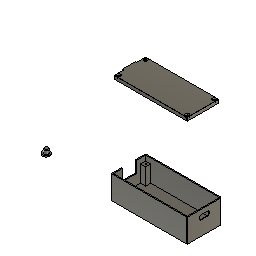
usb-relay (Autodesk Fusion 360 design; units mm, degrees)
Autodesk Fusion 360 part; units mm, degrees
note: some values were not read from the file. Set by a fixed rule: which sketch regions a step uses.
sketch "Skizze1" plane through (0, 0, 0) normal (0, 0, 1) x (1, 0, 0)
  line L0 (0, 0) -> (70, 0)
  line L1 (70, 0) -> (70, 30)
  line L2 (70, 30) -> (0, 30)
  line L3 (0, 30) -> (0, 0)
  circle A0 centre (68, 28) radius 0.7
  circle A1 centre (68, 2) radius 0.7
  circle A2 centre (2, 2) radius 0.7
  circle A3 centre (2, 28) radius 0.7
  line L4 (70, 15) -> (0, 15) construction
  circle A4 centre (36.4, 15) radius 2.5
  dimension "d1" = 70
  dimension "d2" = 30
  dimension "d3" = 1.4
  dimension "d4" = 2
  dimension "d5" = 2
  dimension "d6" = 1.4
  dimension "d7" = 2
  dimension "d8" = 1.4
  dimension "d9" = 2
  dimension "d10" = 1.4
  dimension "d29" = 5
  dimension "d54" = 36.4
  constraint horizontal L0
  constraint vertical L1
  constraint horizontal L2
  constraint vertical L3
  constraint coincident L0.start L3.end
  constraint vertical A0.centre A1.centre
  constraint horizontal A1.centre A2.centre
  constraint vertical A2.centre A3.centre
  constraint horizontal A0.centre A3.centre
  constraint perpendicular L1 L4
  constraint midpoint L3 L4.end
  measures "d1" distance of L0.start L0.end
  measures "d2" distance of L0.start L2.end
  measures "d3" diameter of A0
  measures "d4" distance of L1 A0.centre
  measures "d5" distance of L2 A0.centre
  measures "d6" diameter of A1
  measures "d7" distance of L0 A1.centre
  measures "d8" diameter of A2
  measures "d9" distance of L3 A2.centre
  measures "d10" diameter of A3
  measures "d29" diameter of A4
  measures "d54" distance of L3 A4.centre
extrude "Extrusion1" add sketch "Skizze1" against normal blind 1.6 contours L0 L1 L2 L3 | A4 makes body 1
sketch "Skizze2" plane through (0, 0, 0) normal (-1, 0, 0) x (0, -1, 0)
  line L0 (0, 0) -> (-30, 0)
  line L1 (-30, 0) -> (-30, -1.6)
  line L2 (-30, -1.6) -> (0, -1.6)
  line L3 (0, -1.6) -> (0, 0)
  line L4 (-17.85, 3.3) -> (-12.15, 3.3) construction
  line L5 (-12.15, 0) -> (-17.85, 0)
  arc A0 (-17.85, 3.3) -> (-19.5, 1.65) centre (-17.85, 1.65) ccw construction
  arc A1 (-19.5, 1.65) -> (-17.85, 0) centre (-17.85, 1.65) ccw construction
  arc A2 (-10.5, 1.65) -> (-12.15, 3.3) centre (-12.15, 1.65) ccw construction
  arc A3 (-12.15, 0) -> (-10.5, 1.65) centre (-12.15, 1.65) ccw construction
  arc A4 (-17.85, 3.8) -> (-20, 1.65) centre (-17.85, 1.65) ccw
  arc A5 (-20, 1.65) -> (-17.85, -0.5) centre (-17.85, 1.65) ccw
  line L6 (-12.15, -0.5) -> (-17.85, -0.5)
  arc A6 (-12.15, -0.5) -> (-10, 1.65) centre (-12.15, 1.65) ccw
  arc A7 (-10, 1.65) -> (-12.15, 3.8) centre (-12.15, 1.65) ccw
  line L7 (-17.85, 3.8) -> (-12.15, 3.8)
  point P0 (-19.5, 3.3)
  point P1 (-10.5, 3.3)
  point P2 (-19.5, 0)
  point P3 (-15, 0)
  dimension "d13" = 9
  dimension "d14" = 3.3
  dimension "d15" = 1.65
  dimension "d16" = 1.65
  dimension "d17" = 1.65
  dimension "d18" = 1.65
  dimension "d55" = -0.5
  constraint horizontal L4
  constraint horizontal L5
  constraint coincident P0 L4
  constraint tangent L4 A0
  constraint coincident L5 P3
  constraint coincident P2 L5
  constraint tangent L5 A1
  constraint coincident A0.end A1.start
  constraint coincident P1 L4
  constraint tangent L4 A2
  constraint tangent L5 A3
  constraint coincident A2.start A3.end
  measures "d13" distance of P0 P1
  measures "d14" distance of P0 P2
  measures "d15" radius of A0
  measures "d16" radius of A1
  measures "d17" radius of A2
  measures "d18" radius of A3
extrude "Extrusion2" add sketch "Skizze2" along normal blind 10 contours L0 L5 A5 L6 A6 | L0 L5 A4 A5 A6 A7 L7 bodies 1
sketch "Skizze3" plane through (70, 0, 0) normal (1, 0, 0) x (0, 1, 0)
  line L0 (30, 0) -> (0, 0)
  line L1 (0, 0) -> (0, -1.6)
  line L2 (0, -1.6) -> (30, -1.6)
  line L3 (30, -1.6) -> (30, 0)
  line L4 (8.25, 0) -> (21.75, 0)
  line L5 (21.75, 0) -> (21.75, 6)
  line L6 (21.75, 6) -> (8.25, 6)
  line L7 (8.25, 6) -> (8.25, 0)
  point P0 (15, 0)
  dimension "d21" = 13.5
  dimension "d22" = 6
  constraint horizontal L4
  constraint vertical L5
  constraint horizontal L6
  constraint vertical L7
  constraint midpoint L4 P0
  measures "d21" distance of L4.start L4.end
  measures "d22" distance of L4.start L6.end
extrude "Extrusion3" add sketch "Skizze3" along normal blind 10 separate body contours L0 L4 L5 L6 L7 makes body 2
extrude "Extrusion4" add sketch "Skizze2" against normal blind 2 contours L0 L5 A5 L6 A6 | L0 L5 A4 A5 A6 A7 L7 bodies 1
extrude "Extrusion5" add sketch "Skizze3" against normal blind 2 contours L0 L4 L5 L6 L7 bodies 1 2
extrude "Extrusion6" add sketch "Skizze1" along normal blind 18.5 contours A4 bodies 1
sketch "Skizze4" plane through (0, 0, 0) normal (0, 0, 1) x (1, 0, 0)
  line L0 (116.2217, 0) -> (187.2217, 0)
  line L1 (187.2217, 0) -> (187.2217, 31)
  line L2 (187.2217, 31) -> (116.2217, 31)
  line L3 (116.2217, 31) -> (116.2217, 0)
  line L4 (115.2217, -1) -> (188.2217, -1)
  line L5 (188.2217, -1) -> (188.2217, 32)
  line L6 (188.2217, 32) -> (115.2217, 32)
  line L7 (115.2217, 32) -> (115.2217, -1)
  line L8 (116.2217, 0) -> (121.2217, 0)
  line L9 (121.2217, 0) -> (121.2217, 5)
  line L10 (121.2217, 5) -> (116.2217, 5)
  line L11 (116.2217, 5) -> (116.2217, 0)
  line L12 (187.2217, 0) -> (182.2217, 0)
  line L13 (182.2217, 0) -> (182.2217, 5)
  line L14 (182.2217, 5) -> (187.2217, 5)
  line L15 (187.2217, 5) -> (187.2217, 0)
  line L16 (187.2217, 31) -> (182.2217, 31)
  line L17 (182.2217, 31) -> (182.2217, 26)
  line L18 (182.2217, 26) -> (187.2217, 26)
  line L19 (187.2217, 26) -> (187.2217, 31)
  line L20 (116.2217, 31) -> (121.2217, 31)
  line L21 (121.2217, 31) -> (121.2217, 26)
  line L22 (121.2217, 26) -> (116.2217, 26)
  line L23 (116.2217, 26) -> (116.2217, 31)
  dimension "d32" = 71
  dimension "d33" = 31
  dimension "d34" = 1
  dimension "d39" = 5
  dimension "d40" = 5
  dimension "d41" = 5
  dimension "d42" = 5
  dimension "d43" = 5
  dimension "d44" = 5
  dimension "d45" = 5
  dimension "d46" = 5
  constraint horizontal L0
  constraint vertical L1
  constraint horizontal L2
  constraint vertical L3
  constraint horizontal L8
  constraint vertical L9
  constraint horizontal L10
  constraint vertical L11
  constraint horizontal L12
  constraint vertical L13
  constraint horizontal L14
  constraint vertical L15
  constraint horizontal L16
  constraint vertical L17
  constraint horizontal L18
  constraint vertical L19
  constraint horizontal L20
  constraint vertical L21
  constraint horizontal L22
  constraint vertical L23
  measures "d32" distance of L0.start L0.end
  measures "d33" distance of L0.start L2.end
  measures "d39" distance of L0.start L8.end
  measures "d40" distance of L0.start L10.end
  measures "d41" distance of L0.end L12.end
  measures "d42" distance of L0.end L14.end
  measures "d43" distance of L1.end L16.end
  measures "d44" distance of L1.end L18.end
  measures "d45" distance of L2.end L20.end
  measures "d46" distance of L2.end L22.end
extrude "Extrusion7" add sketch "Skizze4" along normal blind 2 separate body contours L0 L3 L8 L9 L10 L11 | L0 L1 L2 L3 L9 L10 L13 L14 L17 L18 L21 L22 | L0 L1 L12 L13 L14 L15 | L2 L3 L20 L21 L22 L23 | L1 L2 L16 L17 L18 L19 makes body 3
extrude "Extrusion8" add sketch "Skizze4" along normal blind 23 bodies 3
extrude "Extrusion9" add sketch "Skizze4" along normal blind 18 contours L0 L3 L8 L9 L10 L11 | L0 L1 L12 L13 L14 L15 | L2 L3 L20 L21 L22 L23 | L1 L2 L16 L17 L18 L19 bodies 3
extrude "Extrusion10" add sketch "Skizze1" along normal blind 5 contours A0 | A1 | A2 | A3 bodies 1
move_body "Verschieben1" bodies 1 to x (-1, 0, 0) y (0, 1, 0) z (0, 0, -1) at (186.75, 0.5, -6)
move_body "Verschieben2" bodies 1 to x (1, 0, 0) y (0, 1, 0) z (0, 0, 1) at (0, 0, 24)
combine "Kombinieren2" operation cut target body 3 tool bodies 1
sketch "Skizze5" plane through (115.2217, 0, 0) normal (-1, 0, 0) x (0, -1, 0)
  line L0 (-32, 0) -> (1, 0)
  line L1 (1, 0) -> (1, 23)
  line L2 (1, 23) -> (-32, 23)
  line L3 (-32, 23) -> (-32, 0)
  line L4 (-22.25, 18) -> (-8.75, 18)
  line L5 (-8.75, 18) -> (-8.75, 23)
  line L6 (-8.75, 23) -> (-22.25, 23)
  line L7 (-22.25, 23) -> (-22.25, 18)
  line L8 (-8.75, 12) -> (-22.25, 12)
  line L9 (-22.25, 12) -> (-22.25, 18)
  line L10 (-22.25, 18) -> (-8.75, 18)
  line L11 (-8.75, 18) -> (-8.75, 12)
  constraint horizontal L4
  constraint vertical L5
  constraint horizontal L6
  constraint vertical L7
  constraint coincident L2 L5.end
extrude "Extrusion11" cut sketch "Skizze5" against normal blind 5 contours L2 L4 L5 L6 L7 L10 bodies 3
chamfer "Fase1" distance 0.5 angle 45 8 edges at (115.2217, -1, 11.5) (115.2217, 32, 11.5) (115.2217, 15.5, 0) (151.7217, -1, 0) (188.2217, 15.5, 0) (188.2217, -1, 11.5) (188.2217, 32, 11.5) (151.7217, 32, 0) on bodies 3
chamfer "Fase2" distance 0.5 angle 45 4 edges at (187.2217, 10.5, 16.35) (187.2217, 15.5, 14.2) (187.2217, 20.5, 16.35) (187.2217, 15.5, 18.5) on bodies 3
chamfer "Fase3" distance 0.3 angle 45 2 edges at (115.7217, 8.75, 12) (115.7217, 22.25, 12) on bodies 3
ref_plane "Arbeitsebene1" through (0, 0, 105) normal (0, 0, 1) x (1, 0, 0)
sketch "Skizze7" plane through (0, 0, 105) normal (0, 0, 1) x (1, 0, 0)
sketch "Skizze8" plane through (0, 0, 105) normal (0, 0, 1) x (1, 0, 0)
  line L0 (116.2217, 0) -> (187.2217, 0) construction
  line L1 (115.2217, -1) -> (188.2217, -1)
  line L2 (116.2217, 31) -> (116.2217, 0) construction
  line L3 (115.2217, 32) -> (115.2217, -1)
  line L4 (187.2217, 31) -> (116.2217, 31) construction
  line L5 (188.2217, 32) -> (115.2217, 32)
  line L6 (121.2217, 31) -> (121.2217, 26) construction
  line L7 (121.2217, 26) -> (116.2217, 26) construction
  line L8 (121.2217, 5) -> (116.2217, 5) construction
  line L9 (121.2217, 0) -> (121.2217, 5) construction
  line L10 (182.2217, 0) -> (182.2217, 5) construction
  line L11 (182.2217, 5) -> (187.2217, 5) construction
  line L12 (187.2217, 0) -> (187.2217, 31) construction
  line L13 (188.2217, -1) -> (188.2217, 32)
  line L14 (182.2217, 26) -> (187.2217, 26) construction
  line L15 (182.2217, 31) -> (182.2217, 26) construction
  circle A0 centre (184.7217, 2.5) radius 1.2
  circle A1 centre (118.7217, 2.5) radius 1.2
  circle A2 centre (118.7217, 28.5) radius 1.2
  circle A3 centre (184.7217, 28.5) radius 1.2
  circle A4 centre (184.7217, 2.5) radius 1.85
  circle A5 centre (118.7217, 2.5) radius 1.85
  circle A6 centre (118.7217, 28.5) radius 1.85
  circle A7 centre (184.7217, 28.5) radius 1.85
  line L16 (186.5217, 30.7) -> (116.9217, 30.7)
  line L17 (116.5217, 30.3) -> (116.5217, 0.7)
  line L18 (116.9217, 0.3) -> (186.5217, 0.3)
  line L19 (186.9217, 0.7) -> (186.9217, 30.3)
  line L20 (182.2217, 5) -> (121.2217, 5) construction
  line L21 (121.2217, 5) -> (121.2217, 26) construction
  line L22 (121.2217, 26) -> (182.2217, 26) construction
  line L23 (182.2217, 26) -> (182.2217, 5) construction
  arc A8 (186.5217, 0.3) -> (186.9217, 0.7) centre (186.5217, 0.7) ccw
  arc A9 (116.5217, 0.7) -> (116.9217, 0.3) centre (116.9217, 0.7) ccw
  arc A10 (116.9217, 30.7) -> (116.5217, 30.3) centre (116.9217, 30.3) ccw
  arc A11 (186.9217, 30.3) -> (186.5217, 30.7) centre (186.5217, 30.3) ccw
  line L24 (116.2217, 21.95) -> (115.2217, 21.95)
  line L25 (115.2217, 21.95) -> (115.2217, 9.05)
  line L26 (115.2217, 9.05) -> (116.2217, 9.05)
  line L27 (116.2217, 9.05) -> (116.2217, 21.95)
  line L28 (115.2217, 9.05) -> (116.5217, 9.05)
  line L29 (116.5217, 9.05) -> (116.5217, 21.95)
  line L30 (116.5217, 21.95) -> (115.2217, 21.95)
  line L31 (115.2217, 21.95) -> (115.2217, 9.05)
  line L32 (118.8217, 28.4) -> (184.6217, 28.4)
  line L33 (184.6217, 28.4) -> (184.6217, 2.6)
  line L34 (184.6217, 2.6) -> (118.8217, 2.6)
  line L35 (118.8217, 2.6) -> (118.8217, 28.4)
  point P0 (121.2217, 26)
  point P1 (121.2217, 5)
  point P2 (182.2217, 5)
  point P3 (182.2217, 26)
  point P4 (182.2217, 31)
  point P5 (187.2217, 26)
  point P6 (187.2217, 5)
  point P7 (182.2217, 0)
  point P8 (187.2217, 0)
  point P9 (121.2217, 0)
  point P10 (116.2217, 0)
  point P11 (116.2217, 5)
  point P12 (121.2217, 31)
  point P13 (116.2217, 26)
  point P14 (116.2217, 31)
  point P15 (115.2217, 32)
  point P16 (115.2217, -1)
  point P17 (188.2217, -1)
  point P18 (187.2217, 31)
  point P19 (188.2217, 32)
  dimension "d68" = 2.4
  dimension "d69" = 2.4
  dimension "d70" = 2.4
  dimension "d71" = 2.4
  dimension "d72" = 3.7
  dimension "d73" = 3.7
  dimension "d74" = 3.7
  dimension "d75" = 3.7
  dimension "d77" = 0.4
  dimension "d103" = -2.4
  constraint concentric A0 A4
  constraint concentric A1 A5
  constraint concentric A2 A6
  constraint concentric A3 A7
  constraint horizontal L20
  constraint vertical L21
  constraint horizontal L22
  constraint vertical L23
  constraint coincident P0 L6.end
  constraint coincident P2 L10.end
  constraint tangent L18 A8
  constraint tangent L19 A8
  constraint tangent L17 A9
  constraint tangent L18 A9
  constraint equal A8 A9
  constraint tangent L16 A10
  constraint tangent L17 A10
  constraint equal A8 A10
  constraint tangent L16 A11
  constraint tangent L19 A11
  constraint equal A8 A11
  constraint horizontal L28
  constraint vertical L29
  constraint horizontal L30
  constraint vertical L31
  constraint coincident L17 L29.end
  constraint coincident L25.end L26.start
  measures "d68" diameter of A0
  measures "d69" diameter of A1
  measures "d70" diameter of A2
  measures "d71" diameter of A3
  measures "d72" diameter of A4
  measures "d73" diameter of A5
  measures "d74" diameter of A6
  measures "d75" diameter of A7
  measures "d77" radius of A8
extrude "Extrusion13" add sketch "Skizze8" against normal blind 3.2 separate body contours L17 L27 L28 L29 L30 | L16 L17 L18 L19 A8 A9 A10 A11 L29 | A0 A4 L33 L34 | A0 A4 L33 L34 | A3 A7 L32 L33 | A3 A7 L32 L33 | A1 A5 L34 L35 | A1 A5 L34 L35 | A2 A6 L32 L35 | A2 A6 L32 L35 makes body 4
extrude "Extrusion14" cut sketch "Skizze8" against normal blind 1.4 contours A0 A4 L33 L34 | A0 A4 L33 L34 | A3 A7 L32 L33 | A3 A7 L32 L33 | A1 A5 L34 L35 | A1 A5 L34 L35 | A2 A6 L32 L35 | A2 A6 L32 L35 bodies 4
extrude "Extrusion15" add sketch "Skizze8" against normal blind 1.6 contours A4 A5 A6 A7 L32 L33 L34 L35 bodies 4
extrude "Extrusion16" add sketch "Skizze8" against normal blind 5 contours L3 L24 L25 L26 L27 L28 L30 L31 bodies 4
chamfer "Fase5" distance 0.2 angle 45 2 edges at (115.2217, 21.95, 102.5) (115.2217, 9.05, 102.5) on bodies 4
chamfer "Fase6" distance 0.2 angle 45 11 edges at (115.8217, 21.95, 100) (115.3217, 21.85, 100) (115.3217, 9.15, 100) (115.2217, 15.5, 100) (115.8217, 9.05, 100) (115.2217, 15.5, 105) (115.9717, 21.95, 105) (115.9717, 9.05, 105) (116.2217, 21.95, 100.9) (116.2217, 15.5, 100) (116.2217, 9.05, 100.9) on bodies 4
sketch "Skizze9" plane through (0, 0, 0) normal (0, 0, 1) x (1, 0, 0)
  circle A0 centre (44.6609, 6.9568) radius 2.12
  circle A1 centre (44.6609, 6.9568) radius 3.5
  circle A2 centre (44.6609, 6.9568) radius 1.88
  dimension "d89" = 4.24
  dimension "d90" = 7
  dimension "d91" = 3.76
  constraint concentric A0 A1
  constraint concentric A0 A2
  measures "d89" diameter of A0
  measures "d90" diameter of A1
  measures "d91" diameter of A2
extrude "Extrusion17" add sketch "Skizze9" along normal blind 1 separate body contours A1 makes body 5
extrude "Extrusion18" add sketch "Skizze9" along normal blind 5 contours A0 bodies 5
extrude "Extrusion19" add sketch "Skizze9" along normal blind 4 from surface at 1 contours A2 bodies 5
chamfer "Fase7" distance 0.5 angle 45 1 edges at (42.6844, 6.1902, 5) on bodies 5
chamfer "Fase8" distance 0.1 angle 45 9 edges at (151.7217, 30.7, 105) (116.6389, 30.5828, 105) (116.5217, 26.025, 105) (116.5217, 4.975, 105) (116.6389, 0.4172, 105) (151.7217, 0.3, 105) (186.8046, 0.4172, 105) (186.9217, 15.5, 105) (186.8046, 30.5828, 105) on bodies 4
chamfer "Fase9" distance 0.2 angle 45 1 edges at (42.9081, 6.277, 1) on bodies 5
chamfer "Fase10" distance 0.2 angle 45 1 edges at (42.6844, 7.7234, 1) on bodies 5
sketch "Skizze6" plane through (188.2217, 0, 0) normal (1, 0, 0) x (0, 1, 0)
  line L0 (-0.5, 23) -> (-0.5, 0.5)
  line L1 (-0.5, 0.5) -> (31.5, 0.5)
  line L2 (31.5, 0.5) -> (31.5, 23)
  line L3 (31.5, 23) -> (-0.5, 23)
  line L4 (18.35, 14.1) -> (12.65, 14.1)
  arc A0 (12.65, 18.6) -> (12.65, 14.1) centre (12.65, 16.35) ccw
  line L5 (12.65, 18.6) -> (18.35, 18.6)
  arc A1 (18.35, 14.1) -> (18.35, 18.6) centre (18.35, 16.35) ccw
  circle A2 centre (4, 21) radius 1
  circle A3 centre (27, 21) radius 1
  line L6 (0, 18) -> (0, 23)
  line L7 (31, 18) -> (31, 23)
  line L8 (-1, 23) -> (-1, 0.5)
  line L9 (32, 0.5) -> (32, 23)
  dimension "d56" = 2
  dimension "d57" = 2
  dimension "d60" = 2
  dimension "d61" = 5
  dimension "d62" = 5
  constraint horizontal A2.centre A3.centre
  measures "d56" diameter of A2
  measures "d57" diameter of A3
  measures "d60" distance of L3 A2.centre
  measures "d61" distance of A2.centre L8
  measures "d62" distance of A3.centre L9
extrude "Extrusion12" [rolled back] along distance -81 taper angle 0
equation "d6 = d3"
equation "d8 = d3"
equation "d10 = d3"
equation "d39 = d45"
equation "d40 = d45"
equation "d41 = d45"
equation "d42 = d45"
equation "d43 = d45"
equation "d44 = d45"
equation "d46 = d45"
equation "d57 = d56"
equation "d62 = d61"
equation "d69 = d68"
equation "d70 = d68"
equation "d71 = d68"
equation "d73 = d72"
equation "d74 = d72"
equation "d75 = d72"
named bodies: "Case", "Lid", "Button"
